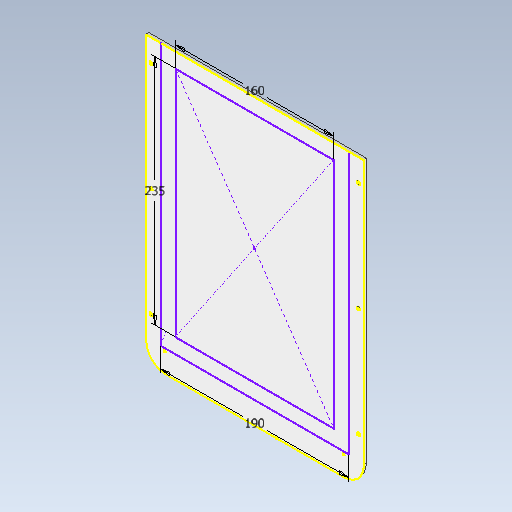
# Autodesk Inventor part: obudowa_zewnetrzna_przod
Saved by Autodesk Inventor 2020 (Build 240168000, 168)
## iProperties
Created: 2020-08-30
Part Number: obudowa_zewnetrzna_przod
Material: ABS Plastic
Document SubType Name: Sheet Metal
Designer: Hesekiel
Density: 1.06 g/cm^3
Appearance: Smooth - White
Sheet Metal Rule: Default
Author: Hesekiel
Autodesk Inventor part; units mm, degrees
ref_plane "YZ Plane" through (0, 0, 0) normal (1, 0, 0) x (0, 1, 0)
ref_plane "XZ Plane" through (0, 0, 0) normal (0, 1, 0) x (-1, 0, 0)
ref_plane "XY Plane" through (0, 0, 0) normal (0, 0, 1) x (1, 0, 0)
sketch "Sketch1" plane through (0, 0, 0) normal (0, 1, 0) x (-1, 0, 0)
  line L0 (-132.5, 287.3805) -> (-122.5, 287.3805)
  line L1 (-132.5, 20) -> (-132.5, 287.3805)
  line L2 (-122.5, 20) -> (-122.5, 287.3805)
  line L3 (77.5, 287.3805) -> (87.5, 287.3805)
  line L4 (77.5, 20) -> (77.5, 287.3805)
  line L5 (87.5, 20) -> (87.5, 287.3805)
  line L6 (82.5, 0) -> (127.5, 0) construction
  line L7 (-132.5, 20) -> (-132.5, 287.3805)
  line L8 (82.5, 45) -> (-127.5, 45)
  line L9 (82.5, 155) -> (-127.5, 155)
  circle A0 centre (-127.5, 265) radius 1.6
  circle A1 centre (-127.5, 155) radius 1.6
  circle A2 centre (-127.5, 45) radius 1.6
  circle A3 centre (82.5, 45) radius 1.6
  circle A4 centre (82.5, 155) radius 1.6
  circle A5 centre (82.5, 265) radius 1.6
  line L10 (-132.5, 287.3805) -> (87.5, 287.3805)
  line L11 (87.5, 287.3805) -> (87.5, 0)
  line L12 (87.5, 0) -> (-132.5, 0)
  line L13 (-132.5, 0) -> (-132.5, 287.3805)
  line L14 (87.5, 0) -> (-132.5, 0)
  line L15 (-132.5, 0) -> (-132.5, -22.8)
  line L16 (-132.5, -22.8) -> (87.5, -22.8)
  line L17 (87.5, -22.8) -> (87.5, 0)
  arc A6 (6, 100) -> (0, 94) centre (6, 94) ccw
  line L18 (0, 0) -> (0, 94)
  line L19 (0, 0) -> (90, 0)
  line L20 (90, 0) -> (90, 94)
  arc A7 (90, 94) -> (84, 100) centre (84, 94) ccw
  line L21 (6, 100) -> (84, 100)
  circle A8 centre (45, 47.3805) radius 11
  circle A9 centre (76.75, 79.1305) radius 5.75
  circle A10 centre (13.25, 15.6305) radius 5.75
  circle A11 centre (76.75, 15.6305) radius 5.75
  circle A12 centre (13.25, 79.1305) radius 5.75
  circle A13 centre (117.5, 135) radius 1.8
  line L22 (112.5, 267.3805) -> (122.5, 267.3805)
  line L23 (112.5, 0) -> (112.5, 267.3805)
  line L24 (112.5, 0) -> (122.5, 0)
  line L25 (122.5, 0) -> (122.5, 267.3805)
  circle A14 centre (117.5, 25) radius 1.8
  circle A15 centre (117.5, 245) radius 1.8
  circle A16 centre (-92.5, 135) radius 1.8
  line L26 (-97.5, 267.3805) -> (-87.5, 267.3805)
  line L27 (-97.5, 0) -> (-97.5, 267.3805)
  line L28 (-97.5, 0) -> (-87.5, 0)
  line L29 (-87.5, 0) -> (-87.5, 267.3805)
  circle A17 centre (-92.5, 245) radius 1.8
  circle A18 centre (-92.5, 25) radius 1.8
  point P0 (-62.5, 0)
  point P1 (52.5, -20)
  dimension "d0" = 45
  dimension "d2" = 110
  dimension "d4" = 3.2
  dimension "d5" = 3.2
  dimension "d6" = 3.2
  dimension "d7" = 3.2
  dimension "d8" = 3.2
  dimension "d9" = 3.2
  dimension "d12" = 22.8
  constraints: 60 end point, 19 centre point, 4 coincident, 4 parallel, 4 point on circle, 3 horizontal, 2 perpendicular, 1 point on line
  measures "d0" distance of L6.start L8.start
  measures "d2" distance of L8.start L9.start
  measures "d4" diameter of A0
  measures "d5" diameter of A1
  measures "d6" diameter of A2
  measures "d7" diameter of A3
  measures "d8" diameter of A4
  measures "d9" diameter of A5
  measures "d12" distance of L15.end L14.end
extrude "Extrusion1" add sketch "Sketch1" along normal blind 3 contours L0 L2 L8 L27 L12 L13 L1 | L10 L4 L9 L29 L26 L27 L2 | L9 L27 L8 L2 | L3 L5 A7 L21 L4 | L27 L26 L29 L9 | L9 L29 L8 L27 | L4 L21 A6 L18 L8 L29 L9 | L27 L8 L29 L12 | L5 L11 L12 L18 L8 A8 L4 A9 L21 A7 | L4 A9 L8 A8 L18 A6 L21 | L29 L8 L18 L12 | A9 L4 | L4 A9 | A8 L8 | L8 A8 | A10 | A11 | A12 | A16 | A17 | A18
fillet "Fillet1" radius 20 2 edges at (132.5, 1.5, 0) (-87.5, 1.5, 0)
sketch "Sketch2" plane through (0, 3, 0) normal (0, 1, 0) x (1, 0, 0)
  arc A0 (-67.5, 0) -> (-87.5, -20) centre (-67.5, -20) ccw projected
  line L0 (-87.5, -20) -> (-87.5, -287.3805) projected
  line L1 (-87.5, -287.3805) -> (132.5, -287.3805) projected
  line L2 (132.5, -287.3805) -> (132.5, -20) projected
  arc A1 (132.5, -20) -> (112.5, 0) centre (112.5, -20) ccw projected
  line L3 (112.5, 0) -> (-67.5, 0) projected
  circle A2 centre (127.5, -155) radius 1.6 projected
  circle A3 centre (127.5, -45) radius 1.6 projected
  circle A4 centre (-82.5, -45) radius 1.6 projected
  circle A5 centre (-82.5, -155) radius 1.6 projected
  circle A6 centre (127.5, -265) radius 1.6 projected
  circle A7 centre (-82.5, -265) radius 1.6 projected
  line L4 (117.5, -287.3805) -> (117.5, -22.3805)
  line L5 (117.5, -22.3805) -> (-72.5, -22.3805)
  line L6 (-72.5, -22.3805) -> (-72.5, -287.3805)
  line L7 (-87.5, -287.3805) -> (132.5, -287.3805) projected
  line L8 (111.1988, -39.9576) -> (117.5, -22.3805) construction
  line L9 (-57.5, -37.3805) -> (102.5, -37.3805)
  line L10 (102.5, -37.3805) -> (102.5, -272.3805)
  line L11 (102.5, -272.3805) -> (-57.5, -272.3805)
  line L12 (-57.5, -272.3805) -> (-57.5, -37.3805)
  line L13 (-57.5, -37.3805) -> (102.5, -272.3805) construction
  line L14 (102.5, -37.3805) -> (-57.5, -272.3805) construction
  point P0 (0, 0)
  point P1 (22.5, -154.8805)
  dimension "d14" = 190
  dimension "d16" = 160
  dimension "d17" = 235
  constraints: 20 end point, 3 parallel, 2 midpoint, 2 point on line, 1 horizontal, 1 perpendicular, 1 point on circle
  measures "d14" distance of L5.end L4.end
  measures "d16" distance of L10.end L11.end
  measures "d17" distance of L9.end L10.end
equation "\"BendRadius\" = Thickness"
equation "\"BendReliefWidth\" = Thickness"
equation "\"BendReliefDepth\" = 0.5 * Thickness"
equation "\"CornerReliefSize\" = 4 * Thickness"
equation "\"MinimumRemnant\" = 2 * Thickness"
equation "\"TransitionRadius\" = BendRadius"
equation "\"JacobiRadiusSize\" = Thickness"
equation "\"GapSize\" = Thickness"
equation "\"Thickness\" = 0.5"
body "Solid1"
